Aufnahme v3_v1 (Autodesk Fusion 360 design; units mm, degrees)
Autodesk Fusion 360 part; units mm, degrees
sketch "Skizze1" plane through (0, 0, 0) normal (0, 0, 1) x (1, 0, 0)
  line L0 (0, 0) -> (80, 0)
  line L1 (80, 0) -> (80, 80)
  line L2 (80, 80) -> (0, 80)
  line L3 (0, 80) -> (0, 0)
  circle A0 centre (40, 40) radius 14
  circle A1 centre (40, 40) radius 16
  dimension "d1" = 28
  dimension "d2" = 32
  constraint horizontal L0
  constraint vertical L1
  constraint horizontal L2
  constraint vertical L3
  constraint coincident L0.start L3.end
  constraint concentric A0 A1
  measures "d1" diameter of A0
  measures "d2" diameter of A1
sketch "Skizze3" plane through (0, 0, 0) normal (0, 0, 1) x (1, 0, 0)
  line L0 (0, 0) -> (10, 50)
  line L1 (10, 50) -> (13, 50)
  line L2 (13, 50) -> (3, 0)
  line L3 (3, 0) -> (0, 0)
  constraint coincident L0.start L3.end
  constraint horizontal L1
  constraint parallel L0 L2
  constraint parallel L1 L3
sketch "Skizze4" plane through (0, 0, 0) normal (0, 0, 1) x (1, 0, 0)
  line L0 (25, 45) -> (25, 0)
  constraint vertical L0
revolve "Drehen2" add sketch "Skizze3" angle 360 about axis through (25, 45, 0) along (0, -1, 0) makes body 1
cylinder "Grundkörper Zylinder1" add diameter 32 height 5 placed x (1, 0, 0) y (0, 0, -1) z (0, 1, 0) at (0, 0, 0) separate body makes body 2
extrude "Extrusion1" add 1 faces at (3.3126, 5, 0.5422) along direction (0, 1, 0) blind 10 on bodies 2 bodies 2
extrude "Extrusion2" cut 1 faces at (3.3126, 15, 0.5422) along direction (0, -1, 0) blind 5 on bodies 2 bodies 2
hole "Bohrung1" at (0, 10, 0) direction (0, -1, 0) diameter 28 depth 15 tip angle 118 countersink diameter 30.8 countersink angle 90 bodies 2
thread "Gewinde1" "ISO Metric Trapezoidal Threads 28.0 TR28x3 7H" major diameter 28.5 minor diameter 25.1575 pitch 3 angle 60 resizes the face on face at (0.6978, 5.7333, 13.9826) on bodies 2
cylinder "Grundkörper Zylinder2" add diameter 32 height 20 placed x (1, 0, 0) y (0, 0, -1) z (0, 1, 0) at (0, 0, 0) separate body makes body 3
cylinder "Grundkörper Zylinder3" cut diameter 30 height -23 placed x (1, 0, 0) y (0, 0, -1) z (0, 1, 0) at (0, 20, 0) bodies 3
move_body "Verschieben1" bodies 2 to x (1, 0, 0) y (0, 1, 0) z (0, 0, 1) at (0, 20, 0)
delete_face "Fläche löschen1" 1 faces at (14.9255, 13.3333, 1.4935) on bodies 3
cylinder "Grundkörper Zylinder4" cut diameter 25.158 height -22 placed x (1, 0, 0) y (0, 0, -1) z (0, 1, 0) at (0, 20, 0) bodies 3
move_face "Fläche verschieben1" by (0, -3, 0) 1 faces at (14.7533, 20, 1.4198) on bodies 3
move_face "Fläche verschieben2" by (0, -3, 0) 1 faces at (14.7883, 20, 1.1082) on bodies 2
copy_body "Körper kopieren/einfügen1" bodies 2 makes body 4
move_body "Verschieben2" bodies 4 to x (-1, 0, 0) y (0, -1, 0) z (0, 0, 1) at (0, 17, 0)
cylinder "Grundkörper Zylinder5" cut diameter 8 height 40 placed x (0, 0, -1) y (0, 1, 0) z (1, 0, 0) at (0, 8.1556, 0) bodies 3
